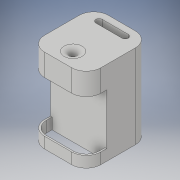
# Autodesk Inventor part: pencil sharpener
Saved by Autodesk Inventor 2017 (Build 210142000, 142)
## iProperties
Created: 2018-03-27
Part Number: pencil sharpener
Material: Generic
Document SubType Name: Modeling
Designer: Braxton
Density: 1 g/cm^3
Appearance: Default
Author: Braxton
Autodesk Inventor part; units mm, degrees
ref_plane "YZ Plane" through (0, 0, 0) normal (1, 0, 0) x (0, 1, 0)
ref_plane "XZ Plane" through (0, 0, 0) normal (0, 1, 0) x (-1, 0, 0)
ref_plane "XY Plane" through (0, 0, 0) normal (0, 0, 1) x (1, 0, 0)
sketch "Sketch1" plane through (0, 0, 0) normal (0, 1, 0) x (-1, 0, 0)
  line L0 (4.0465, 0) -> (4.0465, -4.1391)
  line L1 (1.9447, -6.241) -> (0, -6.241)
  arc A0 (1.9447, -6.241) -> (4.0465, -4.1391) centre (1.9447, -4.1391) ccw
  line L2 (4.0465, 0) -> (0, 0)
  line L3 (0, 0) -> (0, -6.241) construction
  line L4 (-4.0465, 0) -> (-4.0465, -4.1391)
  line L5 (-1.9447, -6.241) -> (0, -6.241)
  arc A1 (-4.0465, -4.1391) -> (-1.9447, -6.241) centre (-1.9447, -4.1391) ccw
  line L6 (-4.0465, 0) -> (0, 0)
  line L7 (0, 0) -> (0, 2.7914) construction
  dimension "d9" = 6.241
  dimension "d11" = 4.0465
  dimension "d12" = 2.1019
  constraints: 16 end point, 4 point on circle, 3 symmetric about line, 2 centre point, 2 collinear, 2 horizontal, 2 perpendicular, 2 tangent, 2 vertical, 1 other
  measures "d9" distance between parallel lines of L2 L1
  measures "d11" distance between parallel lines of L0 L3
  measures "d12" radius of A0
extrude "bace bottom" add sketch "Sketch1" along normal blind 7.3163
sketch "Sketch3" plane through (0, 7.3163, 0) normal (0, 1, 0) x (1, 0, 0)
  line L0 (1.9447, 6.241) -> (-1.9447, 6.241) projected
  line L1 (0, 6.241) -> (0, -3.1186) construction
  line L2 (0, 6.241) -> (-1.9447, 6.241)
  arc A0 (-1.9447, 6.241) -> (-4.0465, 4.1391) centre (-1.9447, 4.1391) ccw projected
  line L3 (-4.0465, 4.1391) -> (-4.0465, -0.825)
  line L4 (-1.9447, -2.9269) -> (0, -2.9269)
  arc A1 (-4.0465, -0.825) -> (-1.9447, -2.9269) centre (-1.9447, -0.825) ccw
  arc A2 (-1.9447, 6.241) -> (-4.0465, 4.1391) centre (-1.9447, 4.1391) ccw
  line L5 (0, 6.241) -> (1.9447, 6.241)
  arc A3 (4.0465, 4.1391) -> (1.9447, 6.241) centre (1.9447, 4.1391) ccw
  line L6 (4.0465, 4.1391) -> (4.0465, -0.825)
  line L7 (1.9447, -2.9269) -> (0, -2.9269)
  arc A4 (1.9447, -2.9269) -> (4.0465, -0.825) centre (1.9447, -0.825) ccw
  constraints: 14 end point, 8 point on circle, 5 symmetric about line, 5 tangent, 4 centre point, 2 vertical, 1 equal radius, 1 horizontal, 1 midpoint, 1 perpendicular, 1 point on line, 2 other
extrude "sharpener top" add sketch "Sketch3" along normal blind 3.175
sketch "Sketch6" plane through (0, 0, 0) normal (1, 0, 0) x (0, 1, 0)
  line L0 (10.4913, 0.825) -> (10.4913, 2.9269) projected
  arc A0 (9.5885, 1.1623) -> (10.4913, 2.0651) centre (9.5885, 2.0651) ccw
  arc A1 (10.4913, -0.5198) -> (9.5885, 0.383) centre (9.5885, -0.5198) ccw construction
  line L1 (10.4913, -4.1391) -> (10.4913, 0.825) projected
  line L2 (9.5885, 0.7726) -> (10.4913, 0.7726)
  line L3 (9.5885, 1.1623) -> (9.5885, 0.7726)
  line L4 (9.5885, 0.383) -> (9.5885, 0.7726) construction
  line L5 (10.4913, 2.0651) -> (10.4913, 0.7726)
  point P0 (0, 0)
  constraints: 8 end point, 4 point on circle, 3 collinear, 3 point on line, 3 tangent, 2 centre point, 2 line through centre, 1 equal radius, 1 perpendicular, 1 vertical
revolve "sharpener hole" cut sketch "Sketch6" angle 360 about axis through (0, 9.5885, 0.7726) along (0, 1, 0)
sketch "Sketch7" plane through (0, 9.5885, 0.7726) normal (0, 1, 0) x (1, 0, 0)
  circle A0 centre (0, 0) radius 0.3897 projected
  circle A1 centre (0, 0) radius 0.3897
  point P0 (0, 0.7726)
  constraints: 1 centre point, 1 coincident
extrude "Extrusion of sharpener hole" cut sketch "Sketch7" against normal blind 1.5875
sketch "Sketch8" plane through (0, 10.4913, 0) normal (0, 1, 0) x (1, 0, 0)
  line L0 (-1.879, 4.8392) -> (1.879, 4.8392) construction
  line L1 (-1.879, 4.3783) -> (1.879, 4.3783)
  line L2 (1.879, 5.3001) -> (-1.879, 5.3001)
  arc A0 (-1.879, 5.3001) -> (-1.879, 4.3783) centre (-1.879, 4.8392) ccw
  arc A1 (1.879, 4.3783) -> (1.879, 5.3001) centre (1.879, 4.8392) ccw
  line L3 (0, 5.3001) -> (0, 4.3783) construction
  line L4 (1.9447, 6.241) -> (-1.9447, 6.241) projected
  line L5 (0, 6.241) -> (0, 6.8422) construction
  point P0 (0, 0)
  point P1 (0, 4.8392)
  constraints: 12 end point, 4 midpoint, 4 point on circle, 4 tangent, 2 centre point, 1 collinear, 1 horizontal, 1 parallel, 1 perpendicular, 1 vertical
extrude "pencil holder" cut sketch "Sketch8" against normal blind 1.5875
sketch "Sketch9" plane through (0, 8.9038, 0) normal (0, 1, 0) x (1, 0, 0)
  line L0 (-1.879, 5.3001) -> (1.879, 5.3001) projected
  line L1 (-0.2544, 5.3001) -> (-1.879, 5.3001)
  line L2 (1.879, 4.3783) -> (-1.879, 4.3783) projected
  line L3 (-1.879, 4.3783) -> (-0.2544, 4.3783)
  line L4 (-0.2544, 5.3001) -> (-0.2544, 4.3783)
  arc A0 (-1.879, 5.3001) -> (-1.879, 4.3783) centre (-1.879, 4.8392) ccw
  line L5 (0, 4.3783) -> (0, 5.3001) construction
  line L6 (0.2544, 5.3001) -> (1.879, 5.3001)
  line L7 (1.879, 4.3783) -> (0.2544, 4.3783)
  line L8 (0.2544, 5.3001) -> (0.2544, 4.3783)
  arc A1 (1.879, 4.3783) -> (1.879, 5.3001) centre (1.879, 4.8392) ccw
  point P0 (0, 0)
  constraints: 14 end point, 4 point on circle, 3 symmetric about line, 2 centre point, 2 midpoint, 2 point on line, 2 tangent, 1 collinear, 1 perpendicular, 1 other
extrude "pencil holder bottom" cut sketch "Sketch9" against normal blind 1.5875 contours L0 L4 L2 A0 | L0 A1 L2 L8
sketch "Sketch10" plane through (0, 0, 0) normal (0, -1, 0) x (1, 0, 0)
  line L0 (-4.0465, 0) -> (4.0465, 0) projected
  line L1 (4.0465, 0.825) -> (4.0465, 0) projected
  line L2 (4.0465, 0) -> (4.0465, 0.825)
  line L3 (-4.0465, 0) -> (-4.0465, 0.825) projected
  line L4 (-4.0465, 0) -> (-4.0465, 0.825)
  arc A0 (-1.9447, 2.9269) -> (-4.0465, 0.825) centre (-1.9447, 0.825) ccw projected
  arc A1 (4.0465, 0.825) -> (1.9447, 2.9269) centre (1.9447, 0.825) ccw projected
  line L5 (-1.9447, 2.9269) -> (1.9447, 2.9269) projected
  line L6 (1.9447, 2.9269) -> (-1.9447, 2.9269)
  arc A2 (-1.9447, 2.9269) -> (-4.0465, 0.825) centre (-1.9447, 0.825) ccw
  arc A3 (4.0465, 0.825) -> (1.9447, 2.9269) centre (1.9447, 0.825) ccw
  arc A4 (1.9447, -6.241) -> (4.0465, -4.1391) centre (1.9447, -4.1391) ccw projected
  line L7 (4.0465, 0) -> (4.0465, -4.1391)
  arc A5 (-4.0465, -4.1391) -> (-1.9447, -6.241) centre (-1.9447, -4.1391) ccw projected
  line L8 (1.9447, -6.241) -> (-1.9447, -6.241)
  line L9 (-4.0465, -4.1391) -> (-4.0465, 0)
  arc A6 (1.9447, -6.241) -> (4.0465, -4.1391) centre (1.9447, -4.1391) ccw
  arc A7 (-4.0465, -4.1391) -> (-1.9447, -6.241) centre (-1.9447, -4.1391) ccw
  line L10 (-3.8061, 0.1518) -> (-3.8061, 0.825)
  arc A8 (-1.9447, 2.6865) -> (-3.8061, 0.825) centre (-1.9447, 0.825) ccw
  line L11 (-1.9447, 2.6865) -> (1.9447, 2.6865)
  arc A9 (3.8061, 0.825) -> (1.9447, 2.6865) centre (1.9447, 0.825) ccw
  line L12 (3.8061, 0.825) -> (3.8061, 0.1877)
  line L13 (3.8061, 0.1877) -> (3.8061, 0)
  line L14 (-3.8061, 0.1518) -> (-3.8061, 0)
  line L15 (-3.8061, 0) -> (3.8061, 0)
  point P0 (0, 0)
  dimension "d24" = 0.2404
  constraints: 24 end point, 12 point on circle, 6 centre point, 6 tangent, 4 perpendicular, 2 collinear, 2 concentric, 2 point on line, 2 vertical, 1 horizontal, 4 other
  measures "d24" distance between parallel lines of L1 L12
extrude "bottom of bace" add sketch "Sketch10" along normal blind 1.5875 contours L3 A0 L5 A1 L1 L0 L13 L12 A9 L11 A8 L10 L14 | L0 L7 A4 L8 A5 L9
body "Solid1"
